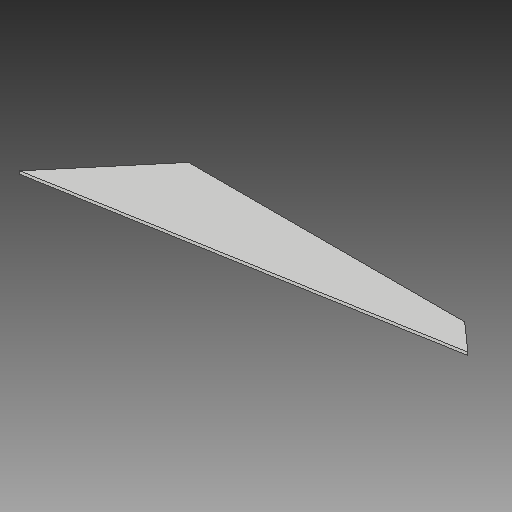
# Autodesk Inventor part: bracket
Saved by Autodesk Inventor 2018.2 (Build 222227000, 227)
## iProperties
Created: 2018-02-26
Part Number: bracket
Material: 一般
Document SubType Name: Modeling
Designer: ku_sk
Density: 1 g/cm^3
Appearance: 既定
Author: ku_sk
Autodesk Inventor part; units mm, degrees
ref_plane "YZ Plane" through (0, 0, 0) normal (1, 0, 0) x (0, 1, 0)
ref_plane "XZ Plane" through (0, 0, 0) normal (0, 1, 0) x (-1, 0, 0)
ref_plane "XY Plane" through (0, 0, 0) normal (0, 0, 1) x (1, 0, 0)
sketch "スケッチ1" plane through (0, 0, 0) normal (0, 1, 0) x (-1, 0, 0)
  line L0 (79.0181, 93.9282) -> (-310.9819, 25.1844)
  line L1 (0, 0) -> (79.0181, 93.9282)
  line L2 (0, 0) -> (-282.639, 0)
  line L3 (-282.639, 0) -> (-310.9819, 25.1844)
  dimension "d1" = 390
  dimension "d2" = 312
  constraints: 8 end point, 1 coincident, 1 horizontal
  measures "d1" horizontal distance of L0.end L0.start
  measures "d2" distance of L0.end L1.start
extrude "押し出し1" add sketch "スケッチ1" along normal mid plane 3
